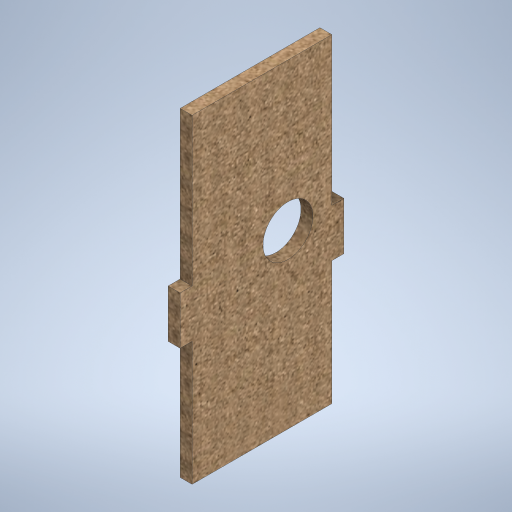
# Autodesk Inventor part: Wheel_Support
Saved by Autodesk Inventor 2024 (Build 280153000, 153)
## iProperties
Created: 2023-11-23
Part Number: Wheel_Support
Material: MDF Tablero de fibras de densidad media
Document SubType Name: Modeling
Designer: marco
Density: 0.8 g/cm^3
Appearance: Cartón - Ondulado
Author: marco
Autodesk Inventor part; units mm, degrees
ref_plane "YZ Plane" through (0, 0, 0) normal (1, 0, 0) x (0, 1, 0)
ref_plane "XZ Plane" through (0, 0, 0) normal (0, 1, 0) x (-1, 0, 0)
ref_plane "XY Plane" through (0, 0, 0) normal (0, 0, 1) x (1, 0, 0)
sketch "Boceto1" plane through (0, 0, 0) normal (1, 0, 0) x (0, 1, 0)
  circle A0 centre (3, -6.5) radius 6.25
  line L0 (-9, 17.5) -> (-9, 20.5)
  line L1 (-9, 20.5) -> (3, 20.5)
  line L2 (3, 20.5) -> (3, 17.5)
  line L3 (3, 17.5) -> (40, 17.5)
  line L4 (40, 17.5) -> (40, -17.5)
  line L5 (40, -17.5) -> (3, -17.5)
  line L6 (3, -17.5) -> (3, -20.5)
  line L7 (3, -20.5) -> (-9, -20.5)
  line L8 (-9, -20.5) -> (-9, -17.5)
  line L9 (-9, -17.5) -> (-40, -17.5)
  line L10 (-40, -17.5) -> (-40, 17.5)
  line L11 (-40, 17.5) -> (-9, 17.5)
  point P0 (0, 0)
  constraints: 24 end point, 1 centre point
extrude "Extrusión1" add sketch "Boceto1" along normal blind 3
